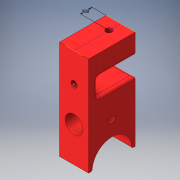
# Autodesk Inventor part: Support Overlay on Gripper Side
Saved by Autodesk Inventor 2016 (Build 200138000, 138)
## iProperties
Created: 2015-07-13
Part Number: Support Overlay on Gripper Side
Material: Aluminum 6061
Document SubType Name: Modeling
Designer: steele
Density: 2.7 g/cm^3
Appearance: Light Red
Mass: 344.296 g
Surface Area: 253.288 cm^2
Volume: 127.517 cm^3
Author: steele
Autodesk Inventor part; units mm, degrees
ref_plane "YZ Plane" through (0, 0, 0) normal (1, 0, 0) x (0, 1, 0)
ref_plane "XZ Plane" through (0, 0, 0) normal (0, 1, 0) x (-1, 0, 0)
ref_plane "XY Plane" through (0, 0, 0) normal (0, 0, 1) x (1, 0, 0)
sketch "Sketch1" plane through (0, 0, 0) normal (0, 0, 1) x (1, 0, 0)
  line L0 (-15.875, -31.75) -> (15.875, -31.75)
  line L1 (15.875, -31.75) -> (15.875, 31.75)
  line L2 (15.875, 31.75) -> (-15.875, 31.75)
  line L3 (-15.875, 31.75) -> (-15.875, -31.75)
  line L4 (-15.875, -31.75) -> (15.875, 31.75) construction
  line L5 (15.875, -31.75) -> (-15.875, 31.75) construction
  point P0 (0, 0)
  dimension "height" = 63.5
  dimension "width" = 31.75
  constraints: 12 end point, 2 midpoint, 2 parallel, 1 horizontal, 1 perpendicular
  measures "height" distance of L2.end L0.start
  measures "width" distance of L1.end L2.end
extrude "Extrusion1" add sketch "Sketch1" along normal blind 50.8
sketch "Sketch2" plane through (0, 0, 0) normal (0, 0, -1) x (-1, 0, 0)
  line L0 (-25.4, -9.525) -> (25.4, -9.525)
  line L1 (25.4, -9.525) -> (25.4, 9.525)
  line L2 (25.4, 9.525) -> (-25.4, 9.525)
  line L3 (-25.4, 9.525) -> (-25.4, -9.525)
  line L4 (-25.4, -9.525) -> (25.4, 9.525) construction
  line L5 (25.4, -9.525) -> (-25.4, 9.525) construction
  point P0 (0, 0)
  dimension "Channel_Width" = 19.05
  constraints: 12 end point, 2 midpoint, 2 parallel, 1 perpendicular
  measures "Channel_Width" distance of L1.end L0.end
extrude "Extrusion2" cut sketch "Sketch2" against normal blind 41.275
sketch "Sketch3" plane through (-15.875, -31.75, 0) normal (0, -1, 0) x (1, 0, 0)
  line L0 (31.75, 41.275) -> (31.75, 0) projected
  line L1 (31.75, 50.8) -> (0, 50.8) projected
  line L2 (31.75, 0) -> (0, 0)
  line L3 (0, 0) -> (0, 50.8)
  line L4 (0, 50.8) -> (31.75, 50.8)
  line L5 (31.75, 50.8) -> (31.75, 0)
  point P0 (15.875, 0)
  constraints: 8 end point, 2 parallel, 1 horizontal, 1 perpendicular
extrude "Extrusion3" add sketch "Sketch3" along normal blind 25.4
sketch "Sketch4" plane through (0, 0, 50.8) normal (0, 0, 1) x (1, 0, 0)
  line L0 (0, 0) -> (0, -57.15) construction
  line L1 (-15.875, -57.15) -> (15.875, -57.15) construction
  line L2 (-15.875, -9.525) -> (-15.875, -57.15) construction
  line L3 (-15.875, -38.1) -> (15.875, -38.1) construction
  circle A0 centre (0, -38.1) radius 9.779
  line L4 (15.875, 31.75) -> (-15.875, 31.75) projected
  dimension "d11" = 19.558
  dimension "Distance_to_Hole" = 69.85
  constraints: 4 end point, 2 midpoint, 1 centre point, 1 horizontal, 1 point on line
  measures "d11" diameter of A0
  measures "Distance_to_Hole" distance between parallel lines of L3 L4
extrude "Extrusion4" cut sketch "Sketch4" against normal through all
sketch "Sketch5" plane through (-15.875, 31.75, 0) normal (-1, 0, 0) x (0, 0, 1)
  line L0 (0, -69.85) -> (50.8, -69.85) construction
  line L1 (50.8, 0) -> (50.8, -88.9) construction
  line L2 (50.8, -88.9) -> (0, -88.9) construction
  line L3 (25.4, -88.9) -> (25.4, -41.275) construction
  line L4 (41.275, -41.275) -> (0, -41.275) construction
  line L5 (0, 0) -> (50.8, 0) projected
  circle A0 centre (25.4, -69.85) radius 3.429
  point P0 (0, -31.75)
  dimension "d19" = 69.85
  dimension "d20" = 6.858
  constraints: 4 end point, 3 point on line, 2 midpoint, 1 centre point, 1 horizontal, 1 vertical
  measures "d19" distance between parallel lines of L0 L5
  measures "d20" diameter of A0
extrude "Extrusion5" cut sketch "Sketch5" against normal through all
sketch "Sketch6" plane through (-15.875, -57.15, 0) normal (0, -1, 0) x (1, 0, 0)
  line L0 (0, 50.8) -> (0, 0) projected
  line L1 (0, 0) -> (31.75, 0) projected
  line L2 (0, 50.8) -> (31.75, 50.8)
  line L3 (31.75, 50.8) -> (31.75, 0)
  line L4 (31.75, 0) -> (0, 0)
  line L5 (0, 0) -> (0, 50.8)
  point P0 (15.875, 0)
  constraints: 8 end point, 2 parallel, 1 horizontal, 1 perpendicular
extrude "Extrusion6" add sketch "Sketch6" along normal blind 19.05
sketch "Sketch7" plane through (15.875, 31.75, 50.8) normal (1, 0, 0) x (0, 0, -1)
  line L0 (50.8, -107.95) -> (0, -107.95) projected
  arc A0 (46.99, -107.95) -> (3.81, -107.95) centre (25.4, -107.95) ccw
  point P0 (50.8, -31.75)
  dimension "d23" = 43.18
  constraints: 2 point on circle, 2 point on line, 1 centre point, 1 midpoint
  measures "d23" diameter of A0
extrude "Extrusion7" cut sketch "Sketch7" against normal through all
sketch "Sketch8" plane through (0, 0, 50.8) normal (0, 0, 1) x (1, 0, 0)
  point P0 (0, 0)
  point P1 (0, 0)
  constraints: 1 coincident
sketch "Sketch11" plane through (-15.875, 31.75, 0) normal (0, 1, 0) x (1, 0, 0)
  line L0 (15.875, 0) -> (15.875, -50.8) construction
  line L1 (25.654, -50.8) -> (6.096, -50.8) construction
  line L2 (31.75, 0) -> (0, 0) construction
  point P0 (15.875, -12.7)
  dimension "d47" = 12.7
  constraints: 2 end point, 1 midpoint, 1 point on line
  measures "d47" distance from line of point (15.875, -12.7) L2
sketch "Sketch12" plane through (0, 0, 50.8) normal (0, 0, 1) x (1, 0, 0)
  point P0 (0, 0)
hole "Hole4" at (0, 0, 50.8) direction (0, 0, -1) diameter 6.7564 depth 9.525
sketch "Sketch13" plane through (-15.875, 31.75, 0) normal (0, 1, 0) x (1, 0, 0)
  point P0 (15.875, -12.7)
hole "Hole6" at (0, 31.75, 12.7) direction (0, -1, 0) diameter 6.7564 depth 22.225
fillet "Fillet1" radius 3.175 10 edges at (-15.875, -9.525, 20.6375) (15.875, -9.525, 20.6375) (0, -9.525, 41.275) (-15.875, 0, 41.275) (15.875, 0, 41.275) (0, 9.525, 0) (0, -9.525, 0) (0, 9.525, 41.275) (-15.875, 9.525, 20.6375) (15.875, 9.525, 20.6375)
fillet "Fillet3" radius 1.5875 2 edges at (0, -76.2, 3.81) (0, -76.2, 46.99)
equation "\"d19\" = Distance_to_Hole"
body "Solid1"
